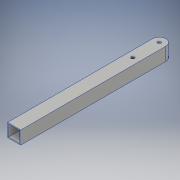
# Autodesk Inventor part: ScissorLiftBarTop
Saved by Autodesk Inventor 2018.3 (Build 223284000, 284)
## iProperties
Created: 2020-01-12
Part Number: ScissorLiftBarTop
Material: Aluminum 6061
Document SubType Name: Modeling
Designer: Cooper
Density: 2.7 g/cm^3
Appearance: Aluminum - Flat
Mass: 227.288 g
Surface Area: 1065.51 cm^2
Volume: 84.1809 cm^3
Author: Cooper
Autodesk Inventor part; units mm, degrees
ref_plane "YZ Plane" through (0, 0, 0) normal (1, 0, 0) x (0, 1, 0)
ref_plane "XZ Plane" through (0, 0, 0) normal (0, 1, 0) x (-1, 0, 0)
ref_plane "XY Plane" through (0, 0, 0) normal (0, 0, 1) x (1, 0, 0)
sketch "Sketch1" plane through (0, 0, 0) normal (0, 0, 1) x (1, 0, 0)
  line L0 (0, 0) -> (25.4, 0)
  line L1 (25.4, 0) -> (25.4, 25.4)
  line L2 (25.4, 25.4) -> (0, 25.4)
  line L3 (0, 25.4) -> (0, 0)
  line L4 (1.5875, 1.5875) -> (23.8125, 1.5875)
  line L5 (23.8125, 1.5875) -> (23.8125, 23.8125)
  line L6 (23.8125, 23.8125) -> (1.5875, 23.8125)
  line L7 (1.5875, 23.8125) -> (1.5875, 1.5875)
  dimension "d0" = 25.4
  dimension "d1" = 25.4
  dimension "d2" = 1.5875
  constraints: 16 end point, 4 parallel, 2 perpendicular, 1 horizontal, 3 other
  measures "d0" distance of L2.end L0.start
  measures "d1" distance of L0.start L0.end
  measures "d2" distance between parallel lines of L6 L2
extrude "Extrusion1" add sketch "Sketch1" along normal blind 558.8
sketch "Sketch3" plane through (0, 25.4, 0) normal (0, 1, 0) x (1, 0, 0)
  line L0 (25.4, 0) -> (0, 0) projected
  line L1 (0, 0) -> (0, -558.8) projected
  line L2 (25.4, -558.8) -> (0, -558.8) projected
  line L3 (25.4, 0) -> (25.4, -558.8) projected
  point P0 (0, 0)
  point P1 (12.7, -279.4)
  dimension "d15" = 279.4
  dimension "d16" = 558.8
  dimension "d17" = 12.7
  measures "d15" distance from line of point (12.7, -279.4) L2
  measures "d16" distance between parallel lines of L0 L2
  measures "d17" distance from line of L1 point (12.7, -279.4)
hole "Hole2" at (12.7, 25.4, 279.4) direction (0, -1, 0) diameter 6.35 end through all clearance for "Flat Head Machine Screw (82)" size "1/4" standard "Ansi Unified Screw Threads"
sketch "Sketch5" plane through (0, 25.4, 0) normal (0, 1, 0) x (1, 0, 0)
  circle A0 centre (12.7, -279.4) radius 3.175 projected
  line L0 (12.7, -279.4) -> (-12.4758, -279.4)
  point P0 (12.7, -228.6)
  point P1 (12.7, -330.2)
  dimension "d25" = 101.6
  constraints: 2 end point, 2 vertical alignment, 1 horizontal, 1 symmetric about line
  measures "d25" distance of point (12.7, -330.2) point (12.7, -228.6)
hole "Hole3" at (12.7, 25.4, 228.6) at (12.7, 25.4, 330.2) direction (0, -1, 0) diameter 6.35 end through all
sketch "Sketch7" plane through (0, 25.4, 0) normal (0, 1, 0) x (1, 0, 0)
  line L0 (0, 0) -> (0, -558.8) projected
  line L1 (25.4, 0) -> (25.4, -558.8) projected
  line L2 (25.4, 0) -> (0, 0) projected
  line L3 (0, 0) -> (25.4, 0) projected
  line L4 (0, -279.4) -> (0, 0)
  line L5 (25.4, 0) -> (25.4, -279.4)
  line L6 (0, 0) -> (25.4, 0)
  arc A0 (25.4, -279.4) -> (0, -279.4) centre (12.7, -279.4) ccw
  dimension "d41" = 279.4
  constraints: 6 end point, 2 midpoint, 2 point on circle, 2 tangent, 1 centre point, 1 collinear, 1 perpendicular
  measures "d41" distance from line of L2 A0.centre
extrude "Extrusion3" cut sketch "Sketch7" against normal blind 25.4
equation "\"d15\" = 0.5 * d16"
body "Solid1"
